Autodesk Inventor part; units mm, degrees
(part 2 of 2)
  arc A185 (-73.6255, 78.4358) -> (-69.8872, 79.8589) centre (-71.7564, 79.1473) ccw
  arc A186 (-48.3486, 90.2723) -> (-70.8652, 77.2723) centre (-59.6069, 83.7723) ccw
  arc A187 (-70.166, 87.2281) -> (-74.0958, 87.6546) centre (-72.1639, 87.137) ccw
  arc A188 (-74.0958, 87.6546) -> (-73.6255, 78.4358) centre (-59.6069, 83.7723) ccw
  arc A189 (-72.1639, 87.137) -> (-71.7564, 79.1473) centre (-59.6069, 83.7723) ccw construction
  line L157 (-56.2422, 96.3293) -> (-49.5268, 91.9816) construction
  arc A190 (-49.5268, 91.9816) -> (-56.2422, 96.3293) centre (-59.6069, 83.7723) ccw construction
  line L158 (-72.1639, 87.137) -> (-71.7564, 79.1473) construction
  arc A191 (-61.9089, 94.5287) -> (-67.7712, 91.1441) centre (-59.6069, 83.7723) ccw
  arc A192 (-55.7246, 98.2612) -> (-57.3201, 94.6447) centre (-56.2422, 96.3293) ccw
  arc A193 (-70.7401, 93.8248) -> (-67.7712, 91.1441) centre (-69.2556, 92.4844) ccw
  arc A194 (-51.0776, 90.7186) -> (-47.976, 93.2445) centre (-49.5268, 91.9816) ccw
  arc A195 (-47.976, 93.2445) -> (-55.7246, 98.2612) centre (-59.6069, 83.7723) ccw
  arc A196 (-61.9089, 94.5287) -> (-62.746, 98.4402) centre (-62.3274, 96.4844) ccw
  arc A197 (-62.3274, 96.4844) -> (-69.2556, 92.4844) centre (-59.6069, 83.7723) ccw construction
  arc A198 (-51.0776, 90.7186) -> (-56.0078, 94.1669) centre (-59.6069, 83.7723) ccw
  line L159 (-59.6069, 83.7723) -> (-56.2422, 96.3293) construction
  line L160 (-49.5268, 91.9816) -> (-59.6069, 83.7723) construction
  arc A199 (-70.4084, 85.8527) -> (-69.8872, 79.8589) centre (-59.6069, 83.7723) ccw
  arc A200 (-48.3486, 90.2723) -> (-70.8652, 77.2723) centre (-59.6069, 83.7723) ccw
  arc A201 (-62.746, 98.4402) -> (-70.7401, 93.8248) centre (-59.6069, 83.7723) ccw
  line L161 (-47.8486, 89.4063) -> (-48.3486, 90.2723)
  line L162 (-44.5958, 83.7723) -> (-44.6069, 83.7916)
  line L163 (-9.3645, 22.75) -> (-40.9647, 77.483)
  arc A202 (-69.5897, -85.1531) -> (-68.9426, -87.5679) centre (-69.2661, -86.3605) ccw projected
  line L164 (66.7941, -94.1669) -> (67.3765, -95.0306)
  line L165 (67.3765, -95.0306) -> (68.1064, -94.6447)
  line L166 (81.1946, -85.8527) -> (81.8311, -86.4062)
  line L167 (81.8311, -86.4062) -> (80.9522, -87.2281)
  line L168 (-70.4084, -85.8527) -> (-70.8652, -86.684)
  line L169 (-70.8652, -86.684) -> (-70.166, -87.2281)
  line L170 (-57.3201, -94.6447) -> (-56.5419, -94.9409)
  line L171 (-56.5419, -94.9409) -> (-56.0078, -94.1669)
  line L172 (-57.3201, 94.6447) -> (-55.1948, 95.1728)
  arc A203 (-55.8113, 93.108) -> (-58.2261, 93.7551) centre (-57.0187, 93.4316) ccw projected
  line L173 (-55.1948, 95.1728) -> (-56.0078, 94.1669)
  line L174 (-70.166, 87.2281) -> (-70.8652, 86.5099)
  line L175 (-70.8652, 86.5099) -> (-70.4084, 85.8527)
  line L176 (66.7941, 94.1669) -> (67.4091, 94.9087)
  line L177 (68.1064, 94.6447) -> (67.4091, 94.9087)
  line L178 (80.9522, 87.2281) -> (81.9652, 86.6432)
  line L179 (81.9652, 86.6432) -> (81.1946, 85.8527)
  point P0 (0, 0)
  point P1 (67.5461, -94.3975)
  point P2 (81.0183, -86.6193)
  point P3 (67.5461, 94.3975)
  point P4 (81.0183, 86.6193)
  point P5 (-72.6069, -83.7723)
  point P6 (-72.6069, -83.7723)
  point P7 (-56.7599, -94.3975)
  point P8 (-70.2321, -86.6193)
  point P9 (-70.2321, 86.6193)
  point P10 (-72.6069, 83.7723)
  point P11 (-56.7599, 94.3975)
  point P12 (-66.1069, 95.0306)
  point P13 (-72.6069, 83.7723)
  dimension "d114" = 8
  dimension "d116" = 35.84
  dimension "d117" = 17.92
  dimension "d118" = 4
  dimension "d119" = 105
  dimension "d120" = 8
  dimension "d121" = 15
  dimension "d122" = 8
  dimension "d123" = 4
  dimension "d124" = 4
  constraints: 191 point on circle, 120 end point, 89 symmetric about line, 75 centre point, 13 tangent, 4 point on line, 2 concentric, 2 equal length, 2 horizontal, 1 coincident, 60 other
  measures "d114" distance of L119.end L120.end
  measures "d116" angle of L119 L120
  measures "d117" angle of L118 L119
  measures "d118" diameter of A130
  measures "d119" angle of L121 L122
  measures "d120" distance of L121.end L123.end
  measures "d121" angle of L125 L126
  measures "d122" distance of L125.end L127.end
  measures "d123" diameter of A135
  measures "d124" diameter of A141
extrude "Extrusion4" add sketch "Sketch4" against normal blind 2.5 contours A184 A182 L116 A3 | A3 L116 A181 A184 | L116 A182 L168 L169 A183 A3 | A3 A183 A181 L116 | A185 A188 A187 A16 | A16 A187 L174 L175 A199 A185 | A174 A172 A173 A3 | A3 A173 A171 A174 | L169 L168 A98 | A179 L170 L171 A177 A178 A3 | A3 A178 A176 A179 | A193 A201 A196 A16 | A16 A196 A191 A193 | A192 A195 A194 A16 | A16 A194 A198 L173 L172 A192 | L172 L173 A103 | A135 A134 L164 L165 A136 A6 | A6 A136 A133 A135 | L165 L164 A87 | A139 A141 A6 L116 | L116 A6 A140 L167 L166 A139 | A130 A129 A131 A6 | A6 A131 A128 A130 | L116 A138 A140 A6 | A6 A141 A138 L116 | L166 L167 A91 | A152 A150 A153 A13 | L176 L177 A83 | A13 A153 L177 L176 A151 A152 | A158 A156 L179 L178 A157 A13 | A13 A157 A155 A158 | A148 A146 A147 A13 | A13 A147 A145 A148 | L178 L179 A81
equation "\"d3\" = d2"
equation "\"d4\" = d2"
equation "\"d22\" = 2 * d21"
equation "\"d45\" = d44"
equation "\"d61\" = 0.5 * d56"
equation "\"d62\" = 0.5 * d53"
equation "\"d69\" = 0.5 * d68"
body "Solid1"
